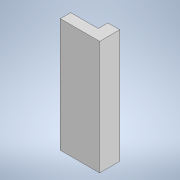
# Autodesk Inventor part: MegaUgolok
Saved by Autodesk Inventor 2020.1 (Build 241239000, 239)
## iProperties
Created: 2023-01-15
Part Number: MegaUgolok
Material: Типовые
Document SubType Name: Modeling
Designer: KirikDK
Density: 1 g/cm^3
Appearance: По умолчанию
Author: KirikDK
Autodesk Inventor part; units mm, degrees
ref_plane "YZ Plane" through (0, 0, 0) normal (1, 0, 0) x (0, 1, 0)
ref_plane "XZ Plane" through (0, 0, 0) normal (0, 1, 0) x (-1, 0, 0)
ref_plane "XY Plane" through (0, 0, 0) normal (0, 0, 1) x (1, 0, 0)
sketch "Эскиз1" plane through (0, 0, 0) normal (0, 1, 0) x (-1, 0, 0)
  line L0 (70.6667, 46) -> (-29.3333, 46)
  line L1 (-29.3333, 46) -> (-29.3333, 19.5)
  line L2 (-29.3333, 19.5) -> (70.6667, 19.5)
  line L3 (70.6667, 19.5) -> (70.6667, 46)
  line L4 (-29.3333, 19.5) -> (0.6667, 19.5)
  line L5 (0.6667, 19.5) -> (0.6667, -5)
  line L6 (0.6667, -5) -> (-29.3333, -5)
  line L7 (-29.3333, -5) -> (-29.3333, 19.5)
  point P0 (0, 0)
  dimension "d0" = 26.5
  dimension "d1" = 100
  dimension "d2" = 30
  dimension "d5" = 51
  constraints: 16 end point, 4 parallel, 2 horizontal, 2 perpendicular
  measures "d0" distance of L2.end L0.start
  measures "d1" distance of L0.start L0.end
  measures "d2" distance of L5.end L6.end
  measures "d5" distance of L0.end L6.end
extrude "Выдавливание1" add sketch "Эскиз1" along normal blind 290
